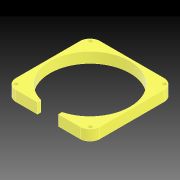
# Autodesk Inventor part: KB33-046-009 - Колпак лидара
Saved by Autodesk Inventor 2020 (Build 240168000, 168)
## iProperties
Created: 2021-08-10
Part Number: KB33-046-009 - Колпак лидара
Material: Типовые
Document SubType Name: Modeling
Designer: Петров Иван
Mass: 16.8694 g
Surface Area: 89.6545 cm^2
Volume: 16.8694 cm^3
Density: 1 g/cm^3
Appearance: Гладкий — желтый
Author: Петров Иван
Autodesk Inventor part; units mm, degrees
ref_plane "YZ Plane" through (0, 0, 0) normal (1, 0, 0) x (0, 1, 0)
ref_plane "XZ Plane" through (0, 0, 0) normal (0, 1, 0) x (-1, 0, 0)
ref_plane "XY Plane" through (0, 0, 0) normal (0, 0, 1) x (1, 0, 0)
sketch "Эскиз1" plane through (0, 0, 0) normal (0, 1, 0) x (-1, 0, 0)
  circle A0 centre (35.3553, 35.3553) radius 2
  circle A1 centre (-35.3553, 35.3553) radius 2
  circle A2 centre (-35.3553, -35.3553) radius 2
  circle A3 centre (35.3553, -35.3553) radius 2
  line L0 (-40, 40) -> (40, 40)
  line L1 (40, 40) -> (40, -40)
  line L2 (40, -40) -> (-40, -40)
  line L3 (-40, -40) -> (-40, 40)
  line L4 (-40, 40) -> (40, -40) construction
  line L5 (40, 40) -> (-40, -40) construction
  point P0 (0, 0)
  dimension "d0" = 4
  dimension "d1" = 50
  dimension "d4" = 360
  dimension "d6" = 80
  dimension "d7" = 80
  constraints: 12 end point, 4 centre point, 2 midpoint, 2 parallel, 1 horizontal, 1 perpendicular, 1 point on line, 9 other
  measures "d0" diameter of A0
  measures "d1" distance of point (0, 0) A0.centre
  measures "d6" distance of L1.end L2.end
  measures "d7" distance of L0.end L1.end
extrude "Выдавливание1" add sketch "Эскиз1" along normal blind 10
sketch "Эскиз3" plane through (0, 10, 0) normal (0, 1, 0) x (1, 0, 0)
  circle A0 centre (0, 0) radius 37.5
  dimension "d16" = 75
  constraints: 1 centre point, 1 coincident
  measures "d16" diameter of A0
extrude "Выдавливание3" cut sketch "Эскиз3" against normal blind 10
thicken "Толщина1" operation add thickness 0.5 both sides no extend neighbours yes toward (0.9972038, 0, 0.0747301) faces at (37.3951, 3.3333, 2.8024)
sketch "Эскиз4" plane through (0, 10, 0) normal (0, 1, 0) x (1, 0, 0)
  line L0 (-10, -42.651) -> (10, -42.651)
  line L1 (10, -42.651) -> (10, -35.651)
  line L2 (10, -35.651) -> (-10, -35.651)
  line L3 (-10, -35.651) -> (-10, -42.651)
  line L4 (-10, -42.651) -> (10, -35.651) construction
  line L5 (10, -42.651) -> (-10, -35.651) construction
  point P0 (0, 0)
  point P1 (0, -39.151)
  dimension "d21" = 20
  dimension "d22" = 7
  constraints: 12 end point, 2 midpoint, 2 parallel, 1 horizontal, 1 perpendicular
  measures "d21" distance of L2.end L1.end
  measures "d22" distance of L1.end L0.end
extrude "Выдавливание4" cut sketch "Эскиз4" against normal blind 10
fillet "Сопряжение1" radius 9.5 4 edges at (-40, 5, 40) (-40, 5, -40) (40, 5, -40) (40, 5, 40)
